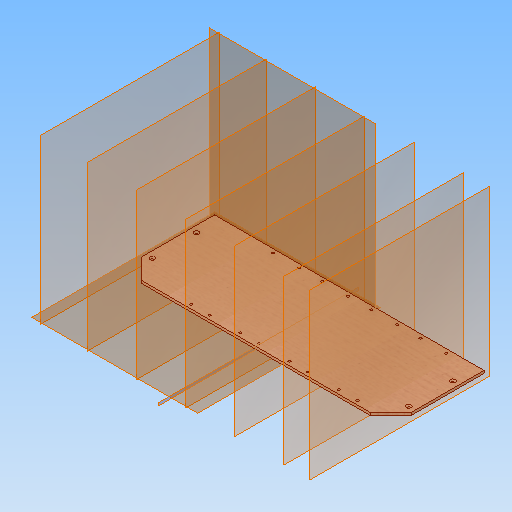
# Autodesk Inventor part: Pancake_Exit Board
Saved by Autodesk Inventor 2018.1 (Build 221171000, 171)
## iProperties
Created: 2019-02-22
Part Number: Pancake_Exit Board
Material: Wood (Oak)
Document SubType Name: Modeling
Designer: James
Density: 0.76 g/cm^3
Appearance: White Oak - Natural Medium Gloss
Mass: 348.215 g
Surface Area: 1914.93 cm^2
Volume: 458.178 cm^3
Author: James
Autodesk Inventor part; units mm, degrees
ref_plane "YZ Plane" through (0, 0, 0) normal (1, 0, 0) x (0, 1, 0)
ref_plane "XZ Plane" through (0, 0, 0) normal (0, 1, 0) x (-1, 0, 0)
ref_plane "XY Plane" through (0, 0, 0) normal (0, 0, 1) x (1, 0, 0)
derived "Pancake_Skeleton.ipt"
ref_plane "Ground" through (0, 0, 0) normal (0, 1, 0) x (-1, 0, 0)
ref_plane "Back" through (0, 0, 0) normal (0, 0, 1) x (1, 0, 0)
ref_plane "LHS" through (0, 0, 0) normal (1, 0, 0) x (0, 1, 0)
ref_plane "Lane 1" through (90, 0, 0) normal (1, 0, 0) x (0, 1, 0)
ref_plane "Lane 2" through (185, 0, 0) normal (1, 0, 0) x (0, 1, 0)
ref_plane "Lane 3" through (280, 0, 0) normal (1, 0, 0) x (0, 1, 0)
ref_plane "Lane 4" through (375, 0, 0) normal (1, 0, 0) x (0, 1, 0)
ref_plane "Lane 5" through (470, 0, 0) normal (1, 0, 0) x (0, 1, 0)
ref_plane "RHS" through (520, 0, 0) normal (1, 0, 0) x (0, 1, 0)
sketch "Sketch1" plane through (0, 0, 0) normal (0, 1, 0) x (-1, 0, 0)
  line L0 (0, -36) -> (0, 216) projected
  line L1 (-520, -36) -> (-520, 216) projected
  line L2 (0, 0) -> (-520, 0)
  line L3 (-520, 0) -> (-520, 180)
  line L4 (-520, 180) -> (0, 180)
  line L5 (0, 180) -> (0, 0)
  dimension "d1" = 180
  constraints: 8 end point, 2 parallel, 1 horizontal, 1 perpendicular, 1 point on line
  measures "d1" distance of L2.end L3.end
extrude "Extrusion1" add sketch "Sketch1" along normal blind 5
sketch "Sketch2" plane through (0, 5, 0) normal (0, 1, 0) x (1, 0, 0)
  line L0 (624, 0) -> (-104, 0) projected
  line L1 (0, 0) -> (0, -180) projected
  line L2 (0, -180) -> (520, -180) projected
  point P0 (12.5, -47.5)
  point P1 (12.5, -132.5)
  dimension "d4" = 47.5
  dimension "d5" = 12.5
  dimension "d6" = 85
  constraints: 1 vertical alignment
  measures "d4" distance from line of L0 point (12.5, -47.5)
  measures "d5" distance from line of L1 point (12.5, -47.5)
  measures "d6" distance of point (12.5, -132.5) point (12.5, -47.5)
hole "Hole1" at (12.5, 5, 47.5) at (12.5, 5, 132.5) direction (0, -1, 0) diameter 4.5 end through all countersink diameter 9.4 countersink angle 90 clearance for "Flat Head Machine Screw" size "M4" standard "Ansi Metric M Profile"
ref_plane "Mid plane" through (260, 0, 0) normal (-1, 0, 0) x (0, 0, 1)
mirror "Mirror1" about plane through (260, 0, 0) normal (-1, 0, 0) of "Hole1"
sketch "Sketch3" plane through (0, 5, 0) normal (0, 1, 0) x (1, 0, 0)
  line L0 (624, 0) -> (-104, 0) projected
  line L1 (0, -180) -> (520, -180) projected
  line L2 (185, 70) -> (185, -420) projected
  line L3 (90, 70) -> (90, -420) projected
  point P0 (0, 0)
  point P1 (120, -7.5)
  point P2 (127, -172.3514)
  point P3 (170, -7.5)
  point P4 (163, -172.3514)
  dimension "d16" = 7.5
  dimension "d45" = 165
  dimension "d46" = 7
  dimension "d47" = 50
  dimension "d48" = 7
  dimension "d49" = 65
  constraints: 2 horizontal alignment
  measures "d16" distance from line of L0 point (120, -7.5)
  measures "d45" distance of point (127, -172.351) point (120, -7.5)
  measures "d46" horizontal distance of point (127, -172.351) point (120, -7.5)
  measures "d47" distance of point (120, -7.5) point (170, -7.5)
  measures "d48" horizontal distance of point (163, -172.351) point (170, -7.5)
  measures "d49" distance from line of point (120, -7.5) L2
hole "Hole2" at (120, 5, 7.5) at (127, 5, 172.3514) at (170, 5, 7.5) at (163, 5, 172.3514) direction (0, -1, 0) diameter 4.5 end through all clearance for "Flat Head Machine Screw" size "M4" standard "Ansi Metric M Profile"
pattern_linear "Rectangular Pattern2" count 4 spacing 95 along (1, 0, 0) of "Hole2"
chamfer "Chamfer2" distance 40 angle 45 2 edges at (520, 2.5, 180) (0, 2.5, 180)
equation "\"d48\" = d46"
body "Solid1"
